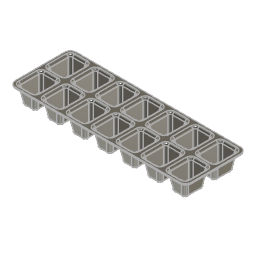
Day 5 - Ice cube Tray (Autodesk Fusion 360 design; units mm, degrees)
part number: 2025-06-16-11-09-07-811
part number: 2025-06-16-11-10-05-177
Autodesk Fusion 360 part; units mm, degrees
sketch "Sketch1" plane through (0, 0, 0) normal (0, 0, 1) x (1, 0, 0) in component "Tray"
  line L0 (0, 0) -> (300, 0)
  line L1 (300, 0) -> (300, 104)
  line L2 (300, 104) -> (0, 104)
  line L3 (0, 104) -> (0, 0)
  dimension "d1" = 300
  dimension "d2" = 104
  constraint horizontal L0
  constraint vertical L1
  constraint horizontal L2
  constraint vertical L3
  constraint coincident L0.start L3.end
  measures "d1" distance of L0.start L0.end
  measures "d2" distance of L0.start L2.end
extrude "Extrude1" add sketch "Sketch1" along normal blind 50 in component "Tray"
sketch "Sketch2" plane through (0, 0, 50) normal (0, 0, 1) x (-1, 0, 0) in component "Tray"
  line L0 (0, -104) -> (0, 0)
  line L1 (0, 0) -> (-300, 0)
  line L2 (-300, 0) -> (-300, -104)
  line L3 (-300, -104) -> (0, -104)
  line L4 (-7, -97) -> (-37, -97)
  line L5 (-37, -97) -> (-37, -57)
  line L6 (-37, -57) -> (-7, -57)
  line L7 (-7, -57) -> (-7, -97)
  dimension "d5" = 30
  dimension "d6" = 40
  dimension "d7" = 7
  dimension "d8" = 7
  constraint horizontal L4
  constraint vertical L5
  constraint horizontal L6
  constraint vertical L7
  measures "d5" distance of L4.start L4.end
  measures "d6" distance of L4.start L6.end
  measures "d7" distance of L3 L4
  measures "d8" distance of L0 L7
extrude "Extrude2" cut sketch "Sketch2" against normal blind 30 draft -10 contours L4 L5 L6 L7 in component "Tray"
fillet "Fillet1" radius 4 5 faces at (35.2367, 81.9034, 40) (25.2367, 58.7633, 40) (8.7633, 72.0966, 40) (18.7633, 95.2367, 40) (18.7633, 81.9034, 20) in component "Tray"
pattern_linear "R-Pattern1" count 7 spacing 42.5 along (1, 0, 0) count 2 spacing 50 along (0, -1, 0) of "Extrude2", "Fillet1" in component "Tray"
shell "Shell1" thickness 2 removed faces 5 at (200, 104, 16.6667) at (300, 34.6667, 16.6667) at (100, 0, 16.6667) at (0, 69.3333, 16.6667) at (100, 69.3333, 0) in component "Tray"
fillet "Fillet2" radius 10 4 edges at (0, 104, 49) (0, 0, 49) (300, 104, 49) (300, 0, 49) in component "Tray"
component "Tray" placed x (1, 0, 0) y (0, 1, 0) z (0, 0, 1) at (0, 0, 0)
